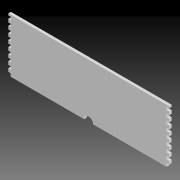
# Autodesk Inventor part: KB33-046-004-017 - Крышка наклонная
Saved by Autodesk Inventor 2020 (Build 240168000, 168)
## iProperties
Created: 2021-06-26
Part Number: KB33-046-004-017 - Крышка наклонная
Material: Типовые
Document SubType Name: Modeling
Designer: Петров Иван
Mass: 90.4818 g
Surface Area: 485.929 cm^2
Volume: 90.4818 cm^3
Density: 1 g/cm^3
Appearance: По умолчанию
Author: Петров Иван
Autodesk Inventor part; units mm, degrees
ref_plane "YZ Plane" through (0, 0, 0) normal (1, 0, 0) x (0, 1, 0)
ref_plane "XZ Plane" through (0, 0, 0) normal (0, 1, 0) x (-1, 0, 0)
ref_plane "XY Plane" through (0, 0, 0) normal (0, 0, 1) x (1, 0, 0)
sketch "Эскиз1" plane through (0, 0, 0) normal (0, 0, 1) x (1, 0, 0)
  line L0 (0, -87.7141) -> (4, -87.7141) projected
  line L1 (4, -87.7141) -> (4, -82.7141) projected
  line L2 (4, -82.7141) -> (0, -82.7141) projected
  line L3 (0, -82.7141) -> (0, -87.7141) projected
  line L4 (4, -77.7141) -> (0, -77.7141) projected
  line L5 (0, -82.7141) -> (0, -77.7141) projected
  line L6 (0, -82.7141) -> (4, -82.7141) projected
  line L7 (4, -77.7141) -> (4, -82.7141) projected
  line L8 (4, -67.7141) -> (0, -67.7141) projected
  line L9 (0, -72.7141) -> (0, -67.7141) projected
  line L10 (0, -72.7141) -> (4, -72.7141) projected
  line L11 (4, -67.7141) -> (4, -72.7141) projected
  line L12 (4, -57.7141) -> (0, -57.7141) projected
  line L13 (0, -62.7141) -> (0, -57.7141) projected
  line L14 (0, -62.7141) -> (4, -62.7141) projected
  line L15 (4, -57.7141) -> (4, -62.7141) projected
  line L16 (4, -47.7141) -> (0, -47.7141) projected
  line L17 (0, -52.7141) -> (0, -47.7141) projected
  line L18 (0, -52.7141) -> (4, -52.7141) projected
  line L19 (4, -47.7141) -> (4, -52.7141) projected
  line L20 (4, -37.7141) -> (0, -37.7141) projected
  line L21 (0, -42.7141) -> (0, -37.7141) projected
  line L22 (0, -42.7141) -> (4, -42.7141) projected
  line L23 (4, -37.7141) -> (4, -42.7141) projected
  line L24 (4, -27.7141) -> (0, -27.7141) projected
  line L25 (0, -32.7141) -> (0, -27.7141) projected
  line L26 (0, -32.7141) -> (4, -32.7141) projected
  line L27 (4, -27.7141) -> (4, -32.7141) projected
  line L28 (4, -17.7141) -> (0, -17.7141) projected
  line L29 (0, -22.7141) -> (0, -17.7141) projected
  line L30 (0, -22.7141) -> (4, -22.7141) projected
  line L31 (4, -17.7141) -> (4, -22.7141) projected
  line L32 (4, -7.7141) -> (0, -7.7141) projected
  line L33 (0, -12.7141) -> (0, -7.7141) projected
  line L34 (0, -12.7141) -> (4, -12.7141) projected
  line L35 (4, -7.7141) -> (4, -12.7141) projected
  line L36 (0, -2.7141) -> (4, -2.7141) projected
  line L37 (4, 0) -> (4, -2.7141) projected
  line L38 (0, 0) -> (4, 0) projected
  line L39 (0, -2.7141) -> (0, 0) projected
  line L40 (-259, -2.7141) -> (-255, -2.7141) projected
  line L41 (-255, 0) -> (-255, -2.7141) projected
  line L42 (-259, 0) -> (-255, 0) projected
  line L43 (-259, -2.7141) -> (-259, 0) projected
  line L44 (-255, -7.7141) -> (-259, -7.7141) projected
  line L45 (-259, -12.7141) -> (-259, -7.7141) projected
  line L46 (-259, -12.7141) -> (-255, -12.7141) projected
  line L47 (-255, -7.7141) -> (-255, -12.7141) projected
  line L48 (-255, -17.7141) -> (-259, -17.7141) projected
  line L49 (-259, -22.7141) -> (-259, -17.7141) projected
  line L50 (-259, -22.7141) -> (-255, -22.7141) projected
  line L51 (-255, -17.7141) -> (-255, -22.7141) projected
  line L52 (-255, -27.7141) -> (-259, -27.7141) projected
  line L53 (-259, -32.7141) -> (-259, -27.7141) projected
  line L54 (-259, -32.7141) -> (-255, -32.7141) projected
  line L55 (-255, -27.7141) -> (-255, -32.7141) projected
  line L56 (-255, -77.7141) -> (-259, -77.7141) projected
  line L57 (-259, -82.7141) -> (-259, -77.7141) projected
  line L58 (-259, -82.7141) -> (-255, -82.7141) projected
  line L59 (-255, -77.7141) -> (-255, -82.7141) projected
  line L60 (-255, -67.7141) -> (-259, -67.7141) projected
  line L61 (-259, -72.7141) -> (-259, -67.7141) projected
  line L62 (-259, -72.7141) -> (-255, -72.7141) projected
  line L63 (-255, -67.7141) -> (-255, -72.7141) projected
  line L64 (-255, -57.7141) -> (-259, -57.7141) projected
  line L65 (-259, -62.7141) -> (-259, -57.7141) projected
  line L66 (-259, -62.7141) -> (-255, -62.7141) projected
  line L67 (-255, -57.7141) -> (-255, -62.7141) projected
  line L68 (-259, -52.7141) -> (-259, -47.7141) projected
  line L69 (-255, -47.7141) -> (-259, -47.7141) projected
  line L70 (-259, -52.7141) -> (-259, -47.7141) projected
  line L71 (-259, -52.7141) -> (-255, -52.7141) projected
  line L72 (-255, -47.7141) -> (-255, -52.7141) projected
  line L73 (-255, -37.7141) -> (-259, -37.7141) projected
  line L74 (-259, -42.7141) -> (-259, -37.7141) projected
  line L75 (-259, -42.7141) -> (-255, -42.7141) projected
  line L76 (-255, -37.7141) -> (-255, -42.7141) projected
  line L77 (-255, -82.7141) -> (-259, -82.7141) projected
  line L78 (-259, -82.7141) -> (-259, -87.7141) projected
  line L79 (-259, -87.7141) -> (-255, -87.7141) projected
  line L80 (-255, -87.7141) -> (-255, -82.7141) projected
  line L81 (-255, 0) -> (0, 0)
  line L82 (0, 0) -> (0, -87.7141)
  line L83 (0, -87.7141) -> (-255, -87.7141)
  line L84 (-255, -87.7141) -> (-255, 0)
  point P0 (-255, -2.7141)
  point P1 (-255, -7.7141)
  point P2 (-255, -12.7141)
  point P3 (-255, -17.7141)
  point P4 (-255, -22.7141)
  point P5 (-255, -27.7141)
  point P6 (-255, -32.7141)
  point P7 (-255, -37.7141)
  point P8 (-255, -42.7141)
  point P9 (-255, -47.7141)
  point P10 (-255, -52.7141)
  point P11 (-255, -57.7141)
  point P12 (-255, -62.7141)
  point P13 (-255, -67.7141)
  point P14 (-255, -72.7141)
  point P15 (-255, -77.7141)
  point P16 (-255, -87.7141)
  constraints: 6 end point, 1 horizontal, 1 parallel, 1 perpendicular, 1 vertical, 3 other
extrude "Выдавливание1" add sketch "Эскиз1" along normal blind 4 contours L83 L80 L59 L84 L63 L67 L72 L76 L55 L51 L47 L41 L81 L39 L82 L33 L29 L25 L21 L17 L13 L9 L5 L3 | L5 L4 L7 L2 | L58 L57 L56 L59 | L9 L8 L11 L10 | L62 L61 L60 L63 | L13 L12 L15 L14 | L66 L65 L64 L67 | L17 L16 L19 L18 | L71 L68 L69 L72 | L21 L20 L23 L22 | L75 L74 L73 L76 | L25 L24 L27 L26 | L54 L53 L52 L55 | L29 L28 L31 L30 | L50 L49 L48 L51 | L33 L32 L35 L34 | L46 L45 L44 L47 | L39 L38 L37 L36 | L40 L43 L42 L41
sketch "Эскиз2" plane through (0, 0, 4) normal (0, 0, 1) x (1, 0, 0)
  line L0 (-255, -87.7141) -> (0, -87.7141) projected
  circle A0 centre (-127.5, -87.7141) radius 7.5
  point P0 (0, 0)
  dimension "d2" = 15
  constraints: 1 centre point, 1 midpoint
  measures "d2" diameter of A0
extrude "Выдавливание2" cut sketch "Эскиз2" against normal blind 4
